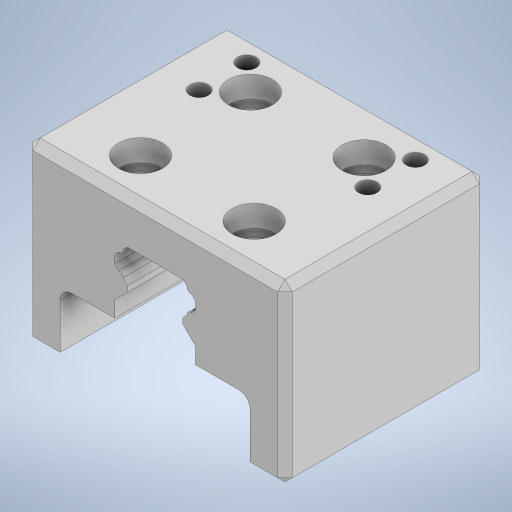
# Autodesk Inventor part: BK12_Spacer
Saved by Autodesk Inventor 2023 (Build 270158000, 158)
## iProperties
Created: 2022-05-04
Part Number: BK12_Spacer
Material: Generic
Document SubType Name: Modeling
Designer: plebbb
Density: 1 g/cm^3
Appearance: Default
Mass: 101.961 g
Surface Area: 235.547 cm^2
Volume: 101.961 cm^3
Author: plebbb
Autodesk Inventor part; units mm, degrees
note: some values were not read from the file. Chosen so that the rebuilt part matches the saved one: second side of "Extrusion1".
ref_plane "YZ Plane" through (0, 0, 0) normal (1, 0, 0) x (0, 1, 0)
ref_plane "XZ Plane" through (0, 0, 0) normal (0, 1, 0) x (-1, 0, 0)
ref_plane "XY Plane" through (0, 0, 0) normal (0, 0, 1) x (1, 0, 0)
sketch "Sketch1" plane through (0, 0, 0) normal (0, 1, 0) x (-1, 0, 0)
  line L0 (0, 0) -> (60, 0) construction
  line L1 (60, 0) -> (60, -25) construction
  line L2 (60, -25) -> (0, -25) construction
  line L3 (0, -25) -> (0, 0) construction
  line L4 (60.5, 0.5) -> (-0.5, 0.5)
  line L5 (-0.5, 0.5) -> (-0.5, -25.5)
  line L6 (-0.5, -25.5) -> (60.5, -25.5)
  line L7 (60.5, -25.5) -> (60.5, 0.5)
  circle A0 centre (53, -19) radius 2.5
  circle A1 centre (7, -19) radius 2.5
  circle A2 centre (7, -6) radius 2.5
  circle A3 centre (53, -6) radius 2.5
  line L8 (53, -19) -> (7, -19) construction
  line L9 (7, -19) -> (7, -6) construction
  line L10 (60.5, 0.5) -> (60.5, 20.5)
  line L11 (60.5, 20.5) -> (-0.5, 20.5)
  line L12 (-0.5, 20.5) -> (-0.5, 0)
  line L13 (89.6876, -43.5705) -> (-21.1545, -43.5705)
  line L14 (-21.1545, -43.5705) -> (-21.1545, 42.1657)
  line L15 (-21.1545, 42.1657) -> (89.6876, 42.1657)
  line L16 (89.6876, 42.1657) -> (89.6876, -43.5705)
  point P0 (30, -19)
  point P1 (30, -25)
  point P2 (7, -12.5)
  point P3 (0, -12.5)
  point P4 (-0.5, 0.5)
  point P5 (-0.5, 0.5)
  dimension "d0" = 25
  dimension "d1" = 60
  dimension "d2" = 0.5
  dimension "d3" = 0.5
  dimension "d4" = 0.5
  dimension "d5" = 0.5
  dimension "d6" = 5
  dimension "d7" = 46
  dimension "d8" = 13
  dimension "d72" = 20
  constraints: 34 end point, 6 parallel, 5 perpendicular, 4 centre point, 4 horizontal, 4 midpoint, 3 equal radius, 3 horizontal alignment, 3 point on line, 3 vertical alignment, 1 vertical
  measures "d0" distance of L0.end L1.end
  measures "d1" distance of L1.end L2.end
  measures "d2" distance between parallel lines of L7 L1
  measures "d3" distance between parallel lines of L5 L3
  measures "d4" distance between parallel lines of L6 L2
  measures "d5" distance between parallel lines of L4 L0
  measures "d6" diameter of A0
  measures "d7" distance of L8.start L8.end
  measures "d8" distance of L8.end L9.end
  measures "d72" distance of L4.start L10.end
sketch "Sketch2" plane through (0, 0, 0) normal (0, 1, 0) x (-1, 0, 0)
  line L0 (-5.4, 29) -> (65.4, 29)
  line L1 (65.4, 29) -> (65.4, -26)
  line L2 (65.4, -26) -> (-5.4, -26)
  line L3 (-5.4, -26) -> (-5.4, 29)
  line L4 (60.5, -25.5) -> (60.5, 0.5) construction
  line L5 (-0.5, 0.5) -> (-0.5, -25.5) construction
  line L6 (-0.5, -25.5) -> (60.5, -25.5) construction
  point P0 (0, 0)
  point P1 (60.5, -12.5)
  point P2 (65.4, 1.5)
  point P3 (30, -26)
  point P4 (30, -25.5)
  point P5 (30, -53.5)
  point P6 (110, 1.5)
  dimension "d9" = 70.8
  dimension "d10" = 55
  dimension "d50" = 35.4
  dimension "d74" = 13.5
  constraints: 8 end point, 4 midpoint, 2 parallel, 1 horizontal, 1 horizontal alignment, 1 perpendicular, 1 vertical alignment
  measures "d9" distance of L1.end L2.end
  measures "d10" distance of L0.end L1.end
  measures "d50" distance from line of L1 point (30, -25.5)
  measures "d74" vertical distance of L1.end point (60.5, -12.5)
extrude "Extrusion1" add sketch "Sketch2" against normal blind 35.4
extrude "Extrusion2" cut sketch "Sketch1" along normal blind 10 and the other way blind 5 contours L7 L6 L5 L4 | L4 L12 L11 L10 | L13 L14 L15 L16
extrude "Extrusion3" cut sketch "Sketch1" along normal blind 10 and the other way blind 30.4 contours A0 | A1 | A2 | A3
sketch "Sketch3" plane through (5.4, -35.4, -26) normal (0, 0, -1) x (1, 0, 0)
  line L0 (-70.8, 0) -> (-70.8, 17.5)
  line L1 (-70.8, 17.5) -> (-61.3, 17.5)
  line L2 (-61.3, 17.5) -> (-61.3, 3.175)
  line L3 (0, 0) -> (0, 17.5)
  line L4 (0, 17.5) -> (-9.5, 17.5)
  line L5 (-9.5, 17.5) -> (-9.5, 3.175)
  arc A0 (-61.3, 3.175) -> (-58.125, 0) centre (-58.125, 3.175) ccw
  arc A1 (-12.675, 0) -> (-9.5, 3.175) centre (-12.675, 3.175) ccw
  line L6 (0, 0) -> (-12.675, 0)
  line L7 (-70.8, -35.4) -> (-70.8, 0) projected
  line L8 (-70.8, 0) -> (0, 0) projected
  line L9 (-58.125, 0) -> (-70.8, 0)
  point P0 (-61.3, 0)
  dimension "d67" = 3.175
  dimension "d68" = 9.5
  dimension "d69" = 17.5
  dimension "d70" = 90
  dimension "d71" = 90
  constraints: 16 end point, 4 point on circle, 3 vertical, 2 centre point, 2 equal length, 2 horizontal, 2 perpendicular, 2 point on line, 2 tangent, 1 equal radius
  measures "d67" radius of A0
  measures "d68" distance of L0.end L1.end
  measures "d69" distance of L0.start L0.end
extrude "Extrusion4" add sketch "Sketch3" against normal up to surface (55 mm away)
sketch "Sketch4" plane through (0, -5, 0) normal (0, 1, 0) x (1, 0, 0)
  circle A0 centre (-45.5, -17.5) radius 3.413
  circle A1 centre (-14.5, -17.5) radius 3.413
  line L0 (-45.5, -17.5) -> (-14.5, -17.5) construction
  line L1 (-65.4, 26) -> (5.4, 26) projected
  line L2 (-45.5, -17.5) -> (-45.5, 12.5) construction
  line L3 (-45.5, 12.5) -> (-14.5, 12.5) construction
  line L4 (-14.5, 12.5) -> (-14.5, -17.5) construction
  circle A2 centre (-45.5, 12.5) radius 3.413
  circle A3 centre (-14.5, 12.5) radius 3.413
  point P0 (-30, -17.5)
  point P1 (-30, 26)
  dimension "d29" = 6.826
  dimension "d78" = 30
  dimension "d79" = 31
  dimension "d80" = 13.5
  constraints: 8 end point, 4 centre point, 3 equal radius, 2 coincident, 2 midpoint, 2 perpendicular, 1 horizontal, 1 vertical, 1 vertical alignment
  measures "d29" diameter of A0
  measures "d78" distance of L0.start L2.end
  measures "d79" distance of L2.end L3.end
  measures "d80" distance from line of L1.start L3
extrude "Extrusion5" cut sketch "Sketch4" against normal blind 36.5125
sketch "Sketch5" plane through (0, -5, 0) normal (0, 1, 0) x (1, 0, 0)
  circle A0 centre (-45.5, -17.5) radius 3.413 construction
  circle A1 centre (-14.5, -17.5) radius 3.413 construction
  circle A2 centre (-14.5, -17.5) radius 6
  circle A3 centre (-45.5, -17.5) radius 6
  circle A4 centre (-45.5, 12.5) radius 6
  circle A5 centre (-14.5, 12.5) radius 6
  circle A6 centre (-14.5, 12.5) radius 3.413 projected
  circle A7 centre (-45.5, 12.5) radius 3.413 projected
  point P0 (0, 0)
  point P1 (-43.1765, -26)
  point P2 (-47.8235, -26)
  point P3 (-12.1765, -26)
  point P4 (-16.8235, -26)
  dimension "d34" = 12
  constraints: 4 centre point, 3 equal radius, 2 concentric, 4 other
  measures "d34" diameter of A3
extrude "Extrusion6" cut sketch "Sketch5" against normal blind 6 contours A2 | A3 | A4 | A5 | A6
sketch "Sketch8" plane through (-52.725, -35.4, 29) normal (0, 0, 1) x (-1, 0, 0)
  line L0 (-22.725, 0) -> (-13.725, 0)
  line L1 (-13.725, 0) -> (-12.725, 1)
  line L2 (-12.725, 1) -> (-12.725, 4)
  line L3 (-12.725, 4) -> (-16.175, 7.45)
  line L4 (-16.175, 7.45) -> (-16.175, 9.8767)
  line L5 (-16.175, 9.8767) -> (-14.9578, 11.0939)
  arc A0 (-13.2458, 12.8058) -> (-14.9578, 11.0939) centre (-12.9761, 10.8241) ccw
  line L6 (-13.2458, 12.8058) -> (-12.725, 13.3267)
  line L7 (-12.725, 13.3267) -> (-12.725, 14.66)
  line L8 (-12.725, 14.66) -> (-13.2458, 15.1808)
  arc A1 (-14.9578, 16.8928) -> (-13.2458, 15.1808) centre (-12.9761, 17.1626) ccw
  line L9 (-14.9578, 16.8928) -> (-15.565, 17.5)
  line L10 (-15.565, 17.5) -> (-22.725, 17.5)
  line L11 (-22.725, 17.5) -> (-22.725, 0) construction
  line L12 (-14.9578, 11.0939) -> (-13.2458, 12.8058) construction
  line L13 (-14.9578, 16.8928) -> (-13.2458, 15.1808) construction
  line L14 (-29.275, 7.45) -> (-29.275, 9.8767)
  line L15 (-29.275, 9.8767) -> (-30.4922, 11.0939)
  line L16 (-30.4922, 11.0939) -> (-32.2042, 12.8058) construction
  arc A2 (-30.4922, 11.0939) -> (-32.2042, 12.8058) centre (-32.4739, 10.8241) ccw
  line L17 (-32.2042, 12.8058) -> (-32.725, 13.3267)
  line L18 (-32.725, 13.3267) -> (-32.725, 14.66)
  line L19 (-32.725, 14.66) -> (-32.2042, 15.1808)
  line L20 (-30.4922, 16.8928) -> (-32.2042, 15.1808) construction
  arc A3 (-32.2042, 15.1808) -> (-30.4922, 16.8928) centre (-32.4739, 17.1626) ccw
  line L21 (-29.885, 17.5) -> (-22.725, 17.5)
  line L22 (-30.4922, 16.8928) -> (-29.885, 17.5)
  line L23 (-32.725, 4) -> (-29.275, 7.45)
  line L24 (-22.725, 0) -> (-31.725, 0)
  line L25 (-32.725, 1) -> (-32.725, 4)
  line L26 (-31.725, 0) -> (-32.725, 1)
  line L27 (-13.725, 0) -> (-12.725, 0)
  line L28 (-12.725, 1) -> (-12.725, 0)
  line L29 (-32.725, 1) -> (-32.725, 0)
  line L30 (-32.725, 0) -> (-31.725, 0)
  line L31 (-13.725, 0) -> (-12.725, -1)
  line L32 (-12.725, -1) -> (-12.725, -4)
  line L33 (-16.175, -7.45) -> (-16.175, -9.8767)
  line L34 (-12.725, -4) -> (-16.175, -7.45)
  line L35 (-12.725, -1) -> (-12.725, 0)
  line L36 (-31.725, 0) -> (-32.725, -1)
  line L37 (-32.725, -4) -> (-29.275, -7.45)
  line L38 (-32.2042, -12.8058) -> (-32.725, -13.3267)
  line L39 (-32.725, -13.3267) -> (-32.725, -14.66)
  line L40 (-29.275, -7.45) -> (-29.275, -9.8767)
  line L41 (-32.725, -14.66) -> (-32.2042, -15.1808)
  line L42 (-30.4922, -11.0939) -> (-32.2042, -12.8058) construction
  arc A4 (-32.2042, -12.8058) -> (-30.4922, -11.0939) centre (-32.4739, -10.8241) ccw
  line L43 (-29.275, -9.8767) -> (-30.4922, -11.0939)
  line L44 (-30.4922, -16.8928) -> (-32.2042, -15.1808) construction
  arc A5 (-30.4922, -16.8928) -> (-32.2042, -15.1808) centre (-32.4739, -17.1626) ccw
  line L45 (-30.4922, -16.8928) -> (-29.885, -17.5)
  line L46 (-29.885, -17.5) -> (-22.725, -17.5)
  line L47 (-22.725, -17.5) -> (-22.725, 0) construction
  line L48 (-32.725, -1) -> (-32.725, 0)
  line L49 (-32.725, -1) -> (-32.725, -4)
  line L50 (-16.175, -9.8767) -> (-14.9578, -11.0939)
  line L51 (-14.9578, -11.0939) -> (-13.2458, -12.8058) construction
  arc A6 (-14.9578, -11.0939) -> (-13.2458, -12.8058) centre (-12.9761, -10.8241) ccw
  line L52 (-13.2458, -12.8058) -> (-12.725, -13.3267)
  line L53 (-12.725, -13.3267) -> (-12.725, -14.66)
  line L54 (-12.725, -14.66) -> (-13.2458, -15.1808)
  line L55 (-15.565, -17.5) -> (-22.725, -17.5)
  line L56 (-14.9578, -16.8928) -> (-13.2458, -15.1808) construction
  arc A7 (-13.2458, -15.1808) -> (-14.9578, -16.8928) centre (-12.9761, -17.1626) ccw
  line L57 (-14.9578, -16.8928) -> (-15.565, -17.5)
  line L58 (-45.45, 0) -> (0, 0) projected
  point P0 (-52.725, -35.4)
  point P1 (-12.725, 2.5)
  point P2 (-32.725, 0.5)
  point P3 (-12.725, -2.5)
  point P4 (-32.725, -0.5)
  dimension "d51" = 1
  dimension "d52" = 3
  dimension "d53" = 135
  dimension "d54" = 2
  dimension "d55" = 3.45
  dimension "d56" = 17.5
  dimension "d57" = 7.16
  dimension "d58" = 2.375
  dimension "d59" = 1.3333
  dimension "d60" = 2.4211
  dimension "d61" = 10
  constraints: 116 end point, 43 symmetric about line, 16 point on circle, 8 centre point, 6 perpendicular, 4 collinear, 3 midpoint, 3 vertical alignment, 2 horizontal, 2 parallel, 2 vertical, 1 equal radius, 6 other
  measures "d51" distance from line of L0 L1.end
  measures "d52" distance of L1.end L2.end
  measures "d53" angle of L2 L3
  measures "d54" radius of A1
  measures "d55" horizontal distance of L4.start L2.end
  measures "d56" distance of L0.start L21.end
  measures "d57" distance of L10.start L21.end
  measures "d58" distance of L12.end L8.end
  measures "d59" distance of L6.end L7.end
  measures "d60" distance of L5.end L12.end
  measures "d61" horizontal distance of L0.start L1.end
extrude "Extrusion9" cut sketch "Sketch8" against normal up to surface (55 mm away) contours L0 L31 L32 L34 L33 L50 A6 L52 L53 L54 A7 L57 L55 L46 L45 A5 L41 L39 L38 A4 L43 L40 L37 L49 L36 L24 | L27 L35 L31 | L36 L48 L30
thicken "Thicken1" operation cut thickness 1 both sides no extend neighbours no toward (-0.7071068, 0.7071068, 0) faces at (-37.7, -29.1, 10.6667) (-40, -32.7333, 10.6667) (-36.55, -26.3322, 10.6667) (-37.3615, -24.7119, 10.6667) (-38.7963, -22.8173, -7.6667) (-39.8264, -22.2469, 10.6667) (-40, -21.1844, -7.6667) (-39.6528, -20.3928, 10.6667) (-39.1967, -20.1597, -7.6667) (-37.3624, -18.1024, 10.6667) (-27.6133, -17.9, -7.6667) (-22.4352, -18.3048, 10.6667) (-21.5595, -19.75, -7.6667) (-20.1736, -20.5664, 10.6667) (-20, -21.6289, -7.6667) (-20.3472, -22.4206, 10.6667) (-22.0096, -23.6233, -7.6667) (-23.0443, -25.1176, -7.6667) (-23.45, -27.1411, 10.6667) (-21.15, -30.25, 10.6667) (-20, -34.0667, 10.6667)
chamfer "Chamfer1" distance 2 angle 45 16 edges at (-65.4, -28.95, -26) (-30, -5, -26) (5.4, -28.95, -26) (-65.4, -5, 1.5) (-65.4, -28.95, 29) (5.4, -5, 1.5) (5.4, -28.95, 29) (-30, -5, 29) (5.4, -52.9, 1.5) (-65.4, -52.9, 1.5) (-60.65, -52.9, 29) (0.65, -52.9, 29) (0.65, -52.9, -26) (-60.65, -52.9, -26) (-55.9, -52.9, 1.5) (-4.1, -52.9, 1.5)
body "Solid1"
